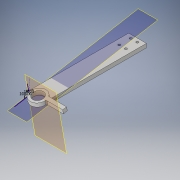
# Autodesk Inventor part: WheelIntakeMotorMount2.0
Saved by Autodesk Inventor 2017 (Build 210142000, 142)
## iProperties
Created: 2017-11-18
Part Number: WheelIntakeMotorMount2.0
Material: Generic
Document SubType Name: Modeling
Designer: User
Density: 1 g/cm^3
Appearance: Default
Author: User
Autodesk Inventor part; units mm, degrees
ref_plane "YZ Plane" through (0, 0, 0) normal (1, 0, 0) x (0, 1, 0)
ref_plane "XZ Plane" through (0, 0, 0) normal (0, 1, 0) x (-1, 0, 0)
ref_plane "XY Plane" through (0, 0, 0) normal (0, 0, 1) x (1, 0, 0)
sketch "Sketch1" plane through (0, 0, 0) normal (1, 0, 0) x (0, 1, 0)
  line L0 (0, 0) -> (21.59, 0)
  line L1 (21.59, 0) -> (21.59, -120.8278)
  line L2 (21.59, -120.8278) -> (0, -120.8278)
  line L3 (0, -120.8278) -> (0, 0)
  dimension "d0" = 21.59
  dimension "d1" = 120.8278
  constraints: 8 end point, 2 parallel, 1 horizontal, 1 perpendicular
  measures "d0" distance of L1.end L2.end
  measures "d1" distance of L0.end L1.end
extrude "Extrusion1" add sketch "Sketch1" along normal blind 4.7625
sketch "Sketch2" plane through (0, 21.59, 0) normal (0, 1, 0) x (1, 0, 0)
  line L0 (0, 0) -> (-3.2071, -18.1884)
  line L1 (0, 0) -> (18.469, 0) construction
  line L2 (0, 0) -> (13.0579, -2.3025)
  line L3 (0, 0) -> (13.2594, 0) construction
  dimension "d4" = 100
  dimension "d24" = 10
  constraints: 8 end point, 2 equal length, 2 horizontal
  measures "d4" angle of L0 L1
  measures "d24" angle of L2 L3
ref_plane "Work Plane1" through (0, 21.59, 0) normal (-0.9848078, 0, -0.1736482) x (-0.1736482, 0, 0.9848078)
sketch "Sketch3" plane through (0, 21.59, 0) normal (-0.9848078, 0, -0.1736482) x (-0.1736482, 0, 0.9848078)
  line L0 (-0.827, 0) -> (-0.827, -21.59) projected
  line L1 (-0.827, -21.59) -> (-119.8192, -21.59) projected
  line L2 (-119.8192, -21.59) -> (-119.8192, 0) projected
  line L3 (-119.8192, 0) -> (-0.827, 0) projected
  line L4 (0, -21.59) -> (0, 0) projected
  line L5 (0, -21.59) -> (-0.827, -21.59) projected
  line L6 (-0.827, 0) -> (-0.827, -21.59) projected
  line L7 (0, 0) -> (-0.827, 0) projected
  line L8 (0, -21.59) -> (0, 0) projected
  circle A0 centre (-0.8636, -10.795) radius 9.525
  dimension "d6" = 21.59
  dimension "d50" = 19.05
  dimension "d51" = 0.8636
  constraints: 1 centre point
  measures "d6" distance of L4.start L4.end
  measures "d50" diameter of A0
  measures "d51" distance from line of L4 A0.centre
extrude "Extrusion2" add sketch "Sketch3" against normal blind 4.7625 contours A0 L4 L0 | L0 A0 | A0 L4
ref_plane "Work Plane3" through (0, 0, 0) normal (-0.1736482, 0, 0.9848078) x (0, 1, 0)
sketch "Sketch9" plane through (4.7625, 0, 0) normal (1, 0, 0) x (0, 0, -1)
  line L0 (0, 21.59) -> (0, 20.3199) projected
  line L1 (0, 0) -> (120.8278, 0) projected
  line L2 (120.8278, 0) -> (120.8278, 21.59) projected
  line L3 (120.8278, 21.59) -> (0, 21.59) projected
  circle A0 centre (109.6528, 10.795) radius 8
  line L4 (102.7246, 14.795) -> (116.581, 14.795)
  line L5 (116.581, 14.795) -> (116.581, 6.795)
  line L6 (116.581, 6.795) -> (102.7246, 6.795)
  line L7 (102.7246, 6.795) -> (102.7246, 14.795)
  ellipse E0 centre (0.0372, 10.795) end of major axis (9.7091, 10.795) minor radius 9.525 (0, 1.2701) -> (0, 20.3199) ccw projected
  line L8 (0, 1.2701) -> (0, 0) projected
  dimension "d34" = 16
  dimension "d35" = 8
  dimension "d36" = 4
  dimension "d37" = 21.59
  dimension "d38" = 10.795
  dimension "d39" = 11.175
  constraints: 8 end point, 3 coincident, 3 point on circle, 2 parallel, 1 centre point, 1 horizontal, 1 perpendicular, 1 point on line, 1 other
  measures "d34" diameter of A0
  measures "d35" distance of L4.end L5.end
  measures "d36" distance from line of L4 A0.centre
  measures "d37" distance of L1.end L2.end
  measures "d38" distance from line of L3 A0.centre
  measures "d39" distance from line of L2 A0.centre
hole "Hole3" at (4.7625, 14.795, -102.7246) at (4.7625, 6.795, -102.7246) at (4.7625, 14.795, -116.581) at (4.7625, 6.795, -116.581) direction (-1, 0, 0) diameter 2.794 end through all
sketch "Sketch11" plane through (4.8401, 10.795, -0.0235) normal (0.9848078, 0, 0.1736482) x (0.1736482, 0, -0.9848078)
  circle A0 centre (0, 0) radius 9.525 projected
  point P0 (-0.8636, -10.795)
hole "Hole4" at (4.8401, 10.795, -0.0235) direction (-0.9848078, 0, -0.1736482) diameter 12.827 end through all
sketch "Sketch12" plane through (4.8401, 10.795, -0.0235) normal (0.9848078, 0, 0.1736482) x (0.1736482, 0, -0.9848078)
  circle A0 centre (0, 0) radius 6.4135 projected
  circle A1 centre (0, 0) radius 9.525 projected
  ellipse E0 centre (114.7733, 4) end of major axis (114.7733, 2.603) minor radius 1.3758 projected
  ellipse E1 centre (101.1274, 4) end of major axis (101.1274, 2.603) minor radius 1.3758 projected
  ellipse E2 centre (101.1274, -4) end of major axis (101.1274, -5.397) minor radius 1.3758 projected
  ellipse E3 centre (114.7733, -4) end of major axis (114.7733, -5.397) minor radius 1.3758 projected
  arc A2 (-0.0366, -9.5249) -> (-0.0366, 9.5249) centre (0, 0) ccw projected
  line L0 (-0.0366, -9.5249) -> (-0.0366, -10.795) projected
  line L1 (-0.0366, -10.795) -> (118.9556, -10.795) projected
  line L2 (118.9556, -10.795) -> (118.9556, 10.795) projected
  line L3 (118.9556, 10.795) -> (-0.0366, 10.795) projected
  line L4 (-0.0366, 10.795) -> (-0.0366, 9.5249) projected
  line L5 (-0.0366, -6.4134) -> (4.7259, -6.4134)
  line L6 (4.7259, -6.4134) -> (4.7259, -29.9338)
  line L7 (4.7259, -29.9338) -> (-0.0366, -29.9338)
  line L8 (-0.0366, -29.9338) -> (-0.0366, -6.4134)
  point P0 (-0.8636, -10.795)
  dimension "d59" = 4.7625
  dimension "d60" = 23.5204
  constraints: 8 end point, 2 parallel, 1 horizontal, 1 perpendicular, 6 other
  measures "d59" distance of L6.end L7.end
  measures "d60" distance of L5.end L6.end
extrude "Extrusion5" add sketch "Sketch12" against normal blind 4.7625 contours L5 L6 A1 L8 | A1 L6 L1 L0 | L1 L6 L7 L8 picked at (2.6364, -7.2637)
equation "\"d36\" = 0.5 * d35"
equation "\"d38\" = 0.5 * d37"
body "Solid1"
